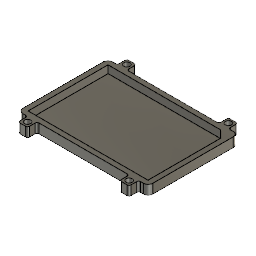
Plate_Lid_96 (Autodesk Fusion 360 design; units mm, degrees)
Autodesk Fusion 360 part; units mm, degrees
sketch "Sketch1" plane through (0, 0, 0) normal (0, 0, 1) x (1, 0, 0)
  line L0 (68.38, -47.235) -> (-68.38, -47.235)
  line L1 (-68.38, -47.235) -> (-68.38, 47.235)
  line L2 (-68.38, 47.235) -> (68.38, 47.235)
  line L3 (68.38, 47.235) -> (68.38, -47.235)
  line L4 (68.38, -47.235) -> (-68.38, 47.235) construction
  line L5 (-68.38, -47.235) -> (68.38, 47.235) construction
  line L6 (-48.38, 47.235) -> (-58.38, 47.235)
  line L7 (-58.38, 47.235) -> (-58.38, 57.235)
  line L8 (-58.38, 57.235) -> (-48.38, 57.235)
  line L9 (-48.38, 57.235) -> (-48.38, 47.235)
  line L10 (-48.38, 47.235) -> (-58.38, 57.235) construction
  line L11 (-58.38, 47.235) -> (-48.38, 57.235) construction
  line L12 (48.38, 57.235) -> (58.38, 57.235)
  line L13 (48.38, 47.235) -> (48.38, 57.235)
  line L14 (58.38, 57.235) -> (58.38, 47.235)
  line L15 (58.38, 47.235) -> (48.38, 47.235)
  line L16 (48.38, -57.235) -> (48.38, -47.235)
  line L17 (48.38, -47.235) -> (58.38, -47.235)
  line L18 (58.38, -47.235) -> (58.38, -57.235)
  line L19 (48.38, -57.235) -> (58.38, -57.235)
  line L20 (-58.38, -57.235) -> (-58.38, -47.235)
  line L21 (-58.38, -47.235) -> (-48.38, -47.235)
  line L22 (-48.38, -47.235) -> (-48.38, -57.235)
  line L23 (-48.38, -57.235) -> (-58.38, -57.235)
  point P0 (-53.38, 52.235)
  dimension "d1" = 136.76
  dimension "d2" = 94.47
  dimension "d3" = 10
  dimension "d4" = 10
  dimension "d6" = 10
  dimension "d7" = 10
  constraint perpendicular L0 L1
  constraint parallel L0 L2
  constraint parallel L1 L3
  constraint horizontal L0
  constraint coincident L4 origin
  constraint coincident L5 origin
  constraint perpendicular L6 L7
  constraint parallel L6 L8
  constraint parallel L7 L9
  constraint horizontal L6
  constraint coincident L10 P0
  constraint coincident L11 P0
  constraint perpendicular L13 L15
  constraint parallel L12 L15
  constraint parallel L13 L14
  constraint horizontal L15
  constraint parallel L16 L18
  constraint perpendicular L18 L19
  constraint perpendicular L20 L23
  constraint parallel L21 L23
  constraint parallel L20 L22
  constraint horizontal L23
  measures "d1" distance of L1.end L2.end
  measures "d2" distance of L0.end L1.end
  measures "d3" distance of L6.end L7.end
  measures "d4" distance of L13.start L12.start
  measures "d6" distance of L16.start L16.end
  measures "d7" distance of L20.start L20.end
extrude "Extrude1" add sketch "Sketch1" along normal blind 10 and the other way blind 0
ref_plane "WorkPlane1" through (0, 0, 10) normal (0, 0, 1) x (1, 0, 0)
sketch "Sketch2" plane through (0, 0, 10) normal (0, 0, 1) x (1, 0, 0)
  line L0 (62.5, -41.5) -> (-62.5, -41.5)
  line L1 (-62.5, -41.5) -> (-62.5, 41.5)
  line L2 (-62.5, 41.5) -> (62.5, 41.5)
  line L3 (62.5, 41.5) -> (62.5, -41.5)
  line L4 (62.5, -41.5) -> (-62.5, 41.5) construction
  line L5 (-62.5, -41.5) -> (62.5, 41.5) construction
  line L6 (-62.5, -41.5) -> (-62.5, 34.9)
  line L7 (62.5, 41.5) -> (-55.8, 41.5)
  line L8 (-62.5, 34.9) -> (-55.8, 41.5)
  dimension "d13" = 125
  dimension "d14" = 83
  dimension "d15" = 76.4
  dimension "d16" = 118.3
  constraint perpendicular L0 L1
  constraint parallel L0 L2
  constraint parallel L1 L3
  constraint horizontal L0
  constraint coincident L4 origin
  constraint coincident L5 origin
  constraint perpendicular L0 L6
  constraint perpendicular L3 L7
  measures "d13" distance of L1.end L2.end
  measures "d14" distance of L0.end L1.end
  measures "d15" distance of L0.end L6.end
  measures "d16" distance of L2.end L7.end
extrude "Extrude2" cut sketch "Sketch2" against normal blind 8 contours L0 L1 L2 L3 L6 L7 L8
ref_plane "WorkPlane2" through (0, 0, 10) normal (0, 0, 1) x (1, 0, 0)
sketch "Sketch3" plane through (0, 0, 10) normal (0, 0, 1) x (1, 0, 0)
  circle A0 centre (-53.3802, 52.2353) radius 3.25
  circle A1 centre (53.38, 52.2349) radius 3.25
  circle A2 centre (53.3799, -52.2347) radius 3.25
  circle A3 centre (-53.3802, -52.2349) radius 3.25
  dimension "d20" = 6.5
  dimension "d21" = 6.5
  dimension "d22" = 6.5
  dimension "d23" = 6.5
  measures "d20" diameter of A0
  measures "d21" diameter of A1
  measures "d22" diameter of A2
  measures "d23" diameter of A3
extrude "Extrude3" cut sketch "Sketch3" against normal blind 10
fillet "Fillet1" radius 5 4 edges at (68.38, -47.235, 5) (68.38, 47.235, 5) (-68.38, -47.235, 5) (-68.38, 47.235, 5)
fillet "Fillet2" radius 2 16 edges at (58.38, -47.235, 5) (58.38, -57.235, 5) (48.38, -57.235, 5) (58.38, 57.235, 5) (-48.38, -47.235, 5) (-48.38, -57.235, 5) (-58.38, -57.235, 5) (-48.38, 57.235, 5) (58.38, 47.235, 5) (-48.38, 47.235, 5) (-58.38, 57.235, 5) (48.38, 57.235, 5) (48.38, 47.235, 5) (-58.38, 47.235, 5) (48.38, -47.235, 5) (-58.38, -47.235, 5)
extrude "Extrude4" add 1 faces at (-18.6, -13.8333, 2) along direction (0, 0, 1) blind 8
ref_plane "WorkPlane3" through (0, 0, 10) normal (0, 0, 1) x (1, 0, 0)
sketch "Sketch4" plane through (0, 0, 10) normal (0, 0, 1) x (1, 0, 0)
  line L0 (63, -42) -> (-63, -42)
  line L1 (-63, -42) -> (-63, 42)
  line L2 (-63, 42) -> (63, 42)
  line L3 (63, 42) -> (63, -42)
  line L4 (63, -42) -> (-63, 42) construction
  line L5 (-63, -42) -> (63, 42) construction
  line L6 (63, -42) -> (63, 34.4)
  line L7 (-63, 42) -> (55.3, 42)
  line L8 (55.3, 42) -> (63, 34.4)
  dimension "d31" = 126
  dimension "d32" = 84
  dimension "d33" = 76.4
  dimension "d34" = 118.3
  constraint perpendicular L0 L1
  constraint parallel L0 L2
  constraint parallel L1 L3
  constraint horizontal L0
  constraint coincident L4 origin
  constraint coincident L5 origin
  constraint perpendicular L0 L6
  constraint perpendicular L1 L7
  measures "d31" distance of L1.end L2.end
  measures "d32" distance of L0.end L1.end
  measures "d33" distance of L0.start L6.end
  measures "d34" distance of L1.end L7.end
extrude "Extrude6" cut sketch "Sketch4" against normal blind 8 contours L0 L1 L2 L3 L6 L7 L8
extrude "Extrude5" cut sketch "Sketch4" against normal blind 8 contours L0 L1 L2 L3 L6 L7 L8
